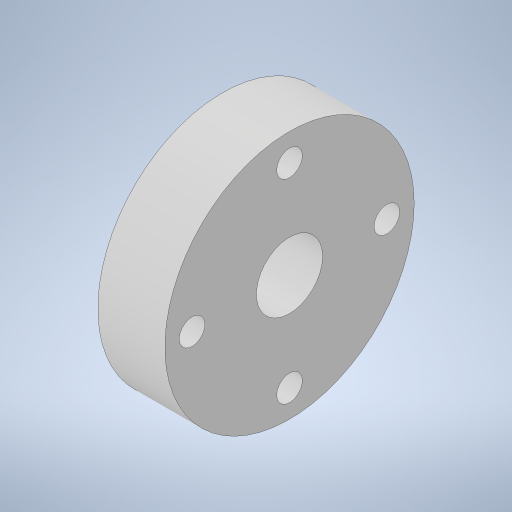
# Autodesk Inventor part: elbow_pully_spacer
Saved by Autodesk Inventor 2024 (Build 280153000, 153)
## iProperties
Created: 2025-08-07
Part Number: elbow_pully_spacer
Material: 一般
Document SubType Name: Modeling
Designer: HosodaLab2
Density: 1 g/cm^3
Appearance: 既定
Author: HosodaLab2
Autodesk Inventor part; units mm, degrees
ref_plane "YZ Plane" through (0, 0, 0) normal (1, 0, 0) x (0, 1, 0)
ref_plane "XZ Plane" through (0, 0, 0) normal (0, 1, 0) x (-1, 0, 0)
ref_plane "XY Plane" through (0, 0, 0) normal (0, 0, 1) x (1, 0, 0)
sketch "スケッチ1" plane through (0, 0, 0) normal (0, 1, 0) x (-1, 0, 0)
  circle A0 centre (0, 0) radius 4.25
  circle A1 centre (0, 0) radius 16
  dimension "d0" = 8.5
  dimension "d1" = 32
  constraints: 2 centre point, 2 coincident
  measures "d0" diameter of A0
  measures "d1" diameter of A1
extrude "押し出し1" add sketch "スケッチ1" along normal blind 8.6
sketch "スケッチ2" plane through (0, 8.6, 0) normal (0, 1, 0) x (1, 0, 0)
  circle A0 centre (0, 0) radius 4.25 construction
  circle A1 centre (0, 0) radius 12.5 construction
  point P0 (-12.5, 0)
  point P1 (0, -12.5)
  point P2 (12.5, 0)
  point P3 (0, 12.5)
  dimension "d4" = 25
  dimension "d7" = 360
  constraints: 1 coincident, 1 horizontal alignment, 7 other
hole "穴1" at (-12.5, 8.6, 0) at (0, 8.6, 12.5) at (12.5, 8.6, 0) at (0, 8.6, -12.5) direction (0, -1, 0) diameter 3.3 end through all
